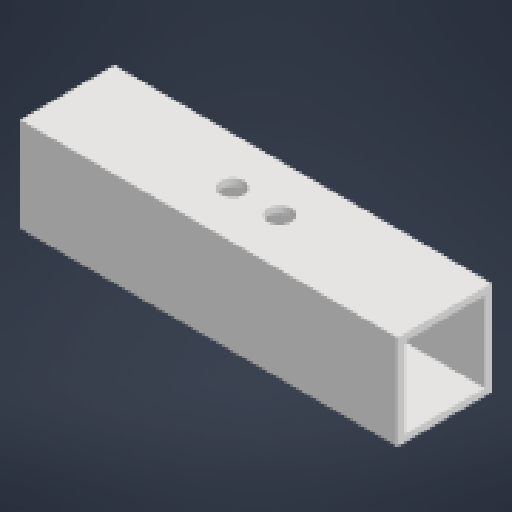
# Autodesk Inventor part: 2
Saved by Autodesk Inventor 2024 (Build 280153000, 153)
## iProperties
Created: 2023-04-17
Part Number: 2
Material: Алюминий 6061
Document SubType Name: Modeling
Designer: user
Density: 2.7 g/cm^3
Appearance: Алюминий — плоский
Author: user
Autodesk Inventor part; units mm, degrees
ref_plane "YZ Plane" through (0, 0, 0) normal (1, 0, 0) x (0, 1, 0)
ref_plane "XZ Plane" through (0, 0, 0) normal (0, 1, 0) x (-1, 0, 0)
ref_plane "XY Plane" through (0, 0, 0) normal (0, 0, 1) x (1, 0, 0)
sketch "Эскиз3" plane through (0, 0, 0) normal (1, 0, 0) x (0, 1, 0)
  line L0 (0, 0) -> (20, 0)
  line L1 (20, 0) -> (20, 20)
  line L2 (20, 20) -> (0, 20)
  line L3 (0, 20) -> (0, 0)
  line L4 (18.5, 18.5) -> (1.5, 18.5)
  line L5 (1.5, 18.5) -> (1.5, 1.5)
  line L6 (1.5, 1.5) -> (18.5, 1.5)
  line L7 (18.5, 1.5) -> (18.5, 18.5)
  point P0 (10, 18.5)
  point P1 (10, 20)
  point P2 (1.5, 10)
  point P3 (0, 10)
  dimension "d2" = 20
  dimension "d3" = 1.5
  constraints: 16 end point, 4 midpoint, 4 parallel, 4 perpendicular, 2 horizontal, 1 horizontal alignment, 1 vertical alignment
  measures "d2" distance of L1.end L2.end
  measures "d3" horizontal distance of L1.end L4.start
extrude "Выдавливание1" add sketch "Эскиз3" along normal blind 50 and the other way blind 30
sketch "Эскиз1" plane through (0, 0, 0) normal (0, 0, 1) x (1, 0, 0)
  circle A0 centre (15, 10) radius 2.5 projected
  circle A1 centre (5, 10) radius 2.5 projected
  point P0 (0, 0)
extrude "Выдавливание2" cut sketch "Эскиз1" along normal through all
sketch "Эскиз4" plane through (-30, 20, 20) normal (0, 1, 0) x (1, 0, 0)
  circle A0 centre (6, 10) radius 2
  circle A1 centre (74, 10) radius 2
  line L0 (80, 20) -> (80, 0) construction
  line L1 (80, 20) -> (0, 20) construction
  line L2 (0, 0) -> (0, 20) construction
  point P0 (30, 20)
  point P1 (80, 10)
  dimension "d10" = 4
  dimension "d11" = 6
  dimension "d12" = 6
  constraints: 2 centre point, 2 horizontal alignment, 1 equal radius, 1 midpoint
  measures "d10" diameter of A0
  measures "d11" horizontal distance of L1.end A0.centre
  measures "d12" horizontal distance of L0.start A1.centre
extrude "Выдавливание3" cut sketch "Эскиз4" against normal through all
